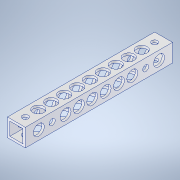
# Autodesk Inventor part: ロボット回転9x9_4
Saved by Autodesk Inventor 2020.3 (Build 243373000, 373)
## iProperties
Created: 2020-07-05
Part Number: ロボット回転9x9_4
Material: アルミニウム 6061
Document SubType Name: Modeling
Designer: totot
Mass: 7.29729 g
Surface Area: 46.6986 cm^2
Volume: 2.7027 cm^3
Density: 2.7 g/cm^3
Appearance: アルミニウム - フラット
Author: totot
Autodesk Inventor part; units mm, degrees
ref_plane "YZ Plane" through (0, 0, 0) normal (1, 0, 0) x (0, 1, 0)
ref_plane "XZ Plane" through (0, 0, 0) normal (0, 1, 0) x (-1, 0, 0)
ref_plane "XY Plane" through (0, 0, 0) normal (0, 0, 1) x (1, 0, 0)
sketch "スケッチ1" plane through (0, 0, 0) normal (0, 0, 1) x (1, 0, 0)
  line L0 (0, 0) -> (9, 0)
  line L1 (9, 0) -> (9, -9)
  line L2 (9, -9) -> (0, -9)
  line L3 (0, -9) -> (0, 0)
  line L4 (1.2, -7.8) -> (7.8, -7.8)
  line L5 (7.8, -7.8) -> (7.8, -1.2)
  line L6 (7.8, -1.2) -> (1.2, -1.2)
  line L7 (1.2, -1.2) -> (1.2, -7.8)
  dimension "d0" = 9
  dimension "d1" = 9
  dimension "d2" = 6.6
  dimension "d3" = 6.6
  dimension "d4" = 1.2
  dimension "d5" = 1.2
  constraints: 16 end point, 4 parallel, 2 horizontal, 2 perpendicular
  measures "d0" distance of L1.end L2.end
  measures "d1" distance of L0.end L1.end
  measures "d2" distance of L6.end L5.end
  measures "d3" distance of L5.end L4.end
  measures "d4" distance between parallel lines of L2 L4
  measures "d5" distance between parallel lines of L7 L3
extrude "押し出し1" add sketch "スケッチ1" along normal blind 74
sketch "スケッチ2" plane through (0, 0, 0) normal (0, 1, 0) x (1, 0, 0)
  line L0 (9, -74) -> (0, -74) projected
  line L1 (9, 0) -> (0, 0) projected
  line L2 (0, 0) -> (0, -74) projected
  point P0 (4.5, -69.5)
  point P1 (4.5, -4.5)
  dimension "d8" = 4.5
  dimension "d9" = 4.5
  dimension "d10" = 4.5
  dimension "d11" = 4.5
  measures "d8" distance from line of point (4.5, -69.5) L0
  measures "d9" distance from line of point (4.5, -4.5) L1
  measures "d10" distance from line of point (4.5, -69.5) L2
  measures "d11" distance from line of L2 point (4.5, -4.5)
hole "穴1" at (4.5, 0, 69.5) at (4.5, 0, 4.5) direction (0, -1, 0) diameter 3 end through all
sketch "スケッチ3" plane through (0, -9, 0) normal (-1, 0, 0) x (0, 0, 1)
  line L0 (0, 9) -> (0, 0) projected
  line L1 (74, 9) -> (74, 0) projected
  line L2 (0, 0) -> (74, 0) projected
  point P0 (60.5, 4.5)
  point P1 (13.5, 4.5)
  dimension "d19" = 13.5
  dimension "d20" = 13.5
  dimension "d21" = 4.5
  dimension "d22" = 4.5
  measures "d19" distance from line of point (13.5, 4.5) L0
  measures "d20" distance from line of point (60.5, 4.5) L1
  measures "d21" distance from line of point (60.5, 4.5) L2
  measures "d22" distance from line of L2 point (13.5, 4.5)
hole "穴2" at (0, -4.5, 60.5) at (0, -4.5, 13.5) direction (1, 0, 0) diameter 3 end through all
sketch "スケッチ4" plane through (0, 0, 0) normal (0, 1, 0) x (1, 0, 0)
  circle A0 centre (4.5, -4.5) radius 1.5 projected
  circle A1 centre (4.5, -69.5) radius 1.5 projected
  circle A2 centre (4.5, -69.5) radius 1.5 projected
  line L0 (4.5, -69.5) -> (4.5, -4.5)
  point P0 (0, 0)
  point P1 (4.5, -63)
  point P2 (4.5, -56.5)
  point P3 (4.5, -50)
  point P4 (4.5, -43.5)
  point P5 (4.5, -37)
  point P6 (4.5, -30.5)
  point P7 (4.5, -24)
  point P8 (4.5, -17.5)
  point P9 (4.5, -11)
  dimension "d30" = 65
  dimension "d31" = 6.5
  dimension "d34" = 6.5
  constraints: 2 end point, 2 vertical, 1 point on line, 8 other
  measures "d30" distance of L0.end A1.centre
  measures "d31" distance of A1.centre point (4.5, -63)
  measures "d34" distance of point (4.5, -63) point (4.5, -56.5)
hole "穴3" at (4.5, 0, 63) at (4.5, 0, 56.5) at (4.5, 0, 50) at (4.5, 0, 43.5) at (4.5, 0, 37) at (4.5, 0, 30.5) at (4.5, 0, 24) at (4.5, 0, 17.5) at (4.5, 0, 11) direction (0, -1, 0) diameter 5.5 end through all
sketch "スケッチ5" plane through (0, -9, 0) normal (-1, 0, 0) x (0, 0, 1)
  line L0 (74, 9) -> (74, 0) projected
  line L1 (0, 9) -> (0, 0) projected
  line L2 (0, 0) -> (74, 0) projected
  circle A0 centre (60.5, 4.5) radius 1.5 projected
  circle A1 centre (13.5, 4.5) radius 1.5 projected
  line L3 (60.5, 4.5) -> (13.5, 4.5)
  point P0 (67.25, 4.5)
  point P1 (6.75, 4.5)
  point P2 (53.7857, 4.5)
  point P3 (47.0714, 4.5)
  point P4 (40.3571, 4.5)
  point P5 (33.6429, 4.5)
  point P6 (26.9286, 4.5)
  point P7 (20.2143, 4.5)
  dimension "d46" = 6.75
  dimension "d47" = 6.75
  dimension "d48" = 4.5
  dimension "d49" = 4.5
  dimension "d50" = 47
  dimension "d51" = 6.7143
  dimension "d54" = 6.7143
  constraints: 2 end point, 2 horizontal, 1 point on line, 5 other
  measures "d46" distance from line of point (67.25, 4.5) L0
  measures "d47" distance from line of point (6.75, 4.5) L1
  measures "d48" distance from line of point (6.75, 4.5) L2
  measures "d49" distance from line of L2 point (67.25, 4.5)
  measures "d50" distance of L3.start L3.end
  measures "d51" distance of L3.start point (53.786, 4.5)
  measures "d54" distance of point (53.786, 4.5) point (47.071, 4.5)
hole "穴4" at (0, -4.5, 67.25) at (0, -4.5, 6.75) at (0, -4.5, 53.7857) at (0, -4.5, 47.0714) at (0, -4.5, 40.3571) at (0, -4.5, 33.6429) at (0, -4.5, 26.9286) at (0, -4.5, 20.2143) direction (1, 0, 0) diameter 5.5 end through all
equation "\"d9\" = d8"
equation "\"d10\" = d8"
equation "\"d11\" = d9"
equation "\"d20\" = d19"
equation "\"d22\" = d21"
equation "\"d31\" = 0.1 * d30"
equation "\"d34\" = d31"
equation "\"d47\" = d46"
equation "\"d49\" = d48"
equation "\"d51\" = 0.142857 * d50"
equation "\"d54\" = d51"
